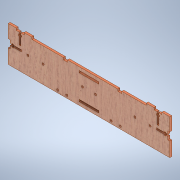
# Autodesk Inventor part: зад
Saved by Autodesk Inventor 2020 (Build 240168000, 168)
## iProperties
Created: 2025-01-17
Part Number: зад
Material: Дерево (орех)
Document SubType Name: ЛистМат
Designer: frozj
Density: 0.55 g/cm^3
Sheet Metal Rule: По умолчанию_мм
Appearance: Орех — натуральный — полированный
Author: frozj
Autodesk Inventor part; units mm, degrees
ref_plane "YZ Plane" through (0, 0, 0) normal (1, 0, 0) x (0, 1, 0)
ref_plane "XZ Plane" through (0, 0, 0) normal (0, 1, 0) x (-1, 0, 0)
ref_plane "XY Plane" through (0, 0, 0) normal (0, 0, 1) x (1, 0, 0)
sketch "Эскиз1" plane through (0, 0, 0) normal (0, 0, 1) x (1, 0, 0)
  line L0 (125, -28.5) -> (-125, -28.5)
  line L1 (-125, -28.5) -> (-125, 28.5)
  line L2 (-125, 28.5) -> (125, 28.5)
  line L3 (125, 28.5) -> (125, -28.5)
  line L4 (125, -28.5) -> (-125, 28.5) construction
  line L5 (-125, -28.5) -> (125, 28.5) construction
  line L6 (-125, 28.5) -> (125, 28.5)
  line L7 (125, 11.5) -> (-125, 11.5)
  line L8 (-125, 11.5) -> (-125, 28.5)
  line L9 (-125, 11.5) -> (125, 11.5)
  line L10 (125, 11.5) -> (125, -8.5)
  line L11 (125, -8.5) -> (-125, -8.5)
  line L12 (-125, -8.5) -> (-125, 11.5)
  line L13 (-125, -8.5) -> (125, -8.5)
  line L14 (125, -8.5) -> (125, -25.5)
  line L15 (125, -25.5) -> (-125, -25.5)
  line L16 (-125, -25.5) -> (-125, -8.5)
  line L17 (-125, 28.5) -> (125, 28.5)
  line L18 (125, 25.5) -> (-125, 25.5)
  line L19 (-125, 25.5) -> (-125, 28.5)
  line L20 (-125, 28.5) -> (-111, 28.5)
  line L21 (-111, 28.5) -> (-111, 25.5)
  line L22 (-111, 25.5) -> (-125, 25.5)
  line L23 (-125, 25.5) -> (-125, 28.5)
  line L24 (-111, 25.5) -> (-99, 25.5)
  line L25 (-99, 25.5) -> (-99, 28.5)
  line L26 (-99, 28.5) -> (-111, 28.5)
  line L27 (-111, 28.5) -> (-111, 25.5)
  line L28 (-99, 28.5) -> (-87, 28.5)
  line L29 (-87, 28.5) -> (-87, 25.5)
  line L30 (-87, 25.5) -> (-99, 25.5)
  line L31 (-99, 25.5) -> (-99, 28.5)
  line L32 (-111, 28.5) -> (-106.35, 28.5)
  line L33 (-106.35, 28.5) -> (-103.65, 28.5)
  line L34 (-103.65, 28.5) -> (-103.65, 8.5)
  line L35 (-103.65, 8.5) -> (-106.35, 8.5)
  line L36 (-106.35, 8.5) -> (-106.35, 28.5)
  line L37 (-106.35, 25.5) -> (-107.45, 25.5)
  line L38 (-107.45, 22.5) -> (-106.35, 22.5)
  line L39 (-106.35, 22.5) -> (-106.35, 25.5)
  line L40 (-107.45, 22.5) -> (-102.55, 22.5)
  line L41 (-102.55, 22.5) -> (-102.55, 20.6)
  line L42 (-102.55, 20.6) -> (-107.45, 20.6)
  line L43 (-107.45, 20.6) -> (-107.45, 22.5)
  line L44 (125, -28.5) -> (125, 28.5)
  line L45 (111, 28.5) -> (111, 25.5)
  line L46 (99, 25.5) -> (99, 28.5)
  line L47 (87, 28.5) -> (87, 25.5)
  line L48 (103.65, 28.5) -> (103.65, 8.5)
  line L49 (103.65, 8.5) -> (106.35, 8.5)
  line L50 (106.35, 8.5) -> (106.35, 28.5)
  line L51 (106.35, 22.5) -> (106.35, 25.5)
  line L52 (107.45, 22.5) -> (102.55, 22.5)
  line L53 (102.55, 22.5) -> (102.55, 20.6)
  line L54 (102.55, 20.6) -> (107.45, 20.6)
  line L55 (107.45, 20.6) -> (107.45, 22.5)
  line L56 (-125, 11.5) -> (-96, 11.5)
  line L57 (-96, 11.5) -> (-96, -8.5)
  line L58 (-96, -8.5) -> (-125, -8.5)
  line L59 (-125, -8.5) -> (-125, 11.5)
  line L60 (-96, -8.5) -> (-67, -8.5)
  line L61 (-67, -8.5) -> (-67, 11.5)
  line L62 (-67, 11.5) -> (-96, 11.5)
  line L63 (-96, 11.5) -> (-96, -8.5)
  line L64 (-96, 1.5) -> (-93, 1.5)
  line L65 (-67, 1.5) -> (-70, 1.5)
  circle A0 centre (-70, 1.5) radius 1.5
  circle A1 centre (-93, 1.5) radius 1.5
  circle A2 centre (70, 1.5) radius 1.5
  circle A3 centre (93, 1.5) radius 1.5
  line L66 (-125, 28.5) -> (-122, 28.5)
  line L67 (-126, 8.5) -> (-125, 28.5)
  line L68 (-126, -3.5) -> (-126, 8.5)
  line L69 (-126, 1.15) -> (-126, 3.85)
  line L70 (-125, 28.5) -> (-123, 28.5)
  line L71 (-123, 28.5) -> (-123, 8.5)
  line L72 (-123, 8.5) -> (-125, 8.5)
  line L73 (-125, 8.5) -> (-125, 28.5)
  line L74 (-123, 8.5) -> (-126, 8.5)
  line L75 (-126, 8.5) -> (-126, -3.5)
  line L76 (-126, -3.5) -> (-123, -3.5)
  line L77 (-123, -3.5) -> (-123, 8.5)
  line L78 (-123, 28.5) -> (-120, 28.5)
  line L79 (-120, 28.5) -> (-120, -3.5)
  line L80 (-120, -3.5) -> (-123, -3.5)
  line L81 (-123, -3.5) -> (-123, 28.5)
  line L82 (-123, 8.5) -> (-120, 8.5)
  line L83 (-120, 8.5) -> (-120, -3.5)
  line L84 (-120, -3.5) -> (-123, -3.5)
  line L85 (-123, -3.5) -> (-123, 8.5)
  line L86 (-123, 8.5) -> (-123, 3.85)
  line L87 (-123, 3.85) -> (-103, 3.85)
  line L88 (-103, 3.85) -> (-103, 1.15)
  line L89 (-103, 1.15) -> (-123, 1.15)
  line L90 (-123, 1.15) -> (-123, 3.85)
  line L91 (-120, 1.15) -> (-117, 1.15)
  line L92 (-117, 1.15) -> (-117, 0.05)
  line L93 (-117, 0.05) -> (-120, 0.05)
  line L94 (-120, 0.05) -> (-120, 1.15)
  line L95 (-117, 0.05) -> (-115.1, 0.05)
  line L96 (-115.1, 0.05) -> (-115.1, 4.95)
  line L97 (-115.1, 4.95) -> (-117, 4.95)
  line L98 (-117, 4.95) -> (-117, 0.05)
  line L99 (123, 3.85) -> (103, 3.85)
  line L100 (103, 3.85) -> (103, 1.15)
  line L101 (103, 1.15) -> (123, 1.15)
  line L102 (120, 1.15) -> (117, 1.15)
  line L103 (117, 0.05) -> (115.1, 0.05)
  line L104 (115.1, 0.05) -> (115.1, 4.95)
  line L105 (115.1, 4.95) -> (117, 4.95)
  line L106 (117, 4.95) -> (117, 0.05)
  line L107 (126, -3.5) -> (123, -3.5)
  line L108 (120, 28.5) -> (120, -3.5)
  line L109 (120, -3.5) -> (123, -3.5)
  line L110 (123, -3.5) -> (123, 28.5)
  line L111 (123, 8.5) -> (125, 8.5)
  line L112 (123, 8.5) -> (120, 8.5)
  line L113 (-123, -3.5) -> (-125, -3.5)
  line L114 (-125, -3.5) -> (-125, -28.5)
  line L115 (-125, -28.5) -> (-123, -28.5)
  line L116 (-123, -28.5) -> (-123, -3.5)
  line L117 (123, -3.5) -> (125, -3.5)
  line L118 (125, -3.5) -> (125, -28.5)
  line L119 (125, -28.5) -> (123, -28.5)
  line L120 (123, -28.5) -> (123, -3.5)
  line L121 (-67, -8.5) -> (-14.5, -8.5)
  line L122 (-14.5, -28.5) -> (-67, -28.5)
  line L123 (-40.75, -28.5) -> (-33.75, -28.5)
  circle A4 centre (-33.75, -21.5) radius 1.5
  circle A5 centre (-47.75, -21.5) radius 1.5
  circle A6 centre (33.75, -21.5) radius 1.5
  circle A7 centre (47.75, -21.5) radius 1.5
  line L124 (-33.75, -25.5) -> (-47.75, -25.5)
  line L125 (-47.75, -28.5) -> (-33.75, -28.5)
  line L126 (-40.75, -28.5) -> (-28.75, -28.5)
  line L127 (-28.75, -28.5) -> (-28.75, -25.5)
  line L128 (-28.75, -25.5) -> (-40.75, -25.5)
  line L129 (-40.75, -28.5) -> (-52.75, -28.5)
  line L130 (-52.75, -28.5) -> (-52.75, -25.5)
  line L131 (-52.75, -25.5) -> (-40.75, -25.5)
  line L132 (-40.75, -25.5) -> (-40.75, -28.5)
  line L133 (28.75, -28.5) -> (28.75, -25.5)
  line L134 (52.75, -28.5) -> (52.75, -25.5)
  line L135 (52.5, -17.5) -> (-52.5, -17.5)
  line L136 (-52.5, -17.5) -> (-52.5, 17.5)
  line L137 (-52.5, 17.5) -> (52.5, 17.5)
  line L138 (52.5, 17.5) -> (52.5, -17.5)
  line L139 (52.5, -17.5) -> (-52.5, 17.5) construction
  line L140 (-52.5, -17.5) -> (52.5, 17.5) construction
  line L141 (15, 14.5) -> (-15, 14.5)
  line L142 (-15, 14.5) -> (-15, 20.5)
  line L143 (-15, 20.5) -> (15, 20.5)
  line L144 (15, 20.5) -> (15, 14.5)
  line L145 (15, 14.5) -> (-15, 20.5) construction
  line L146 (-15, 14.5) -> (15, 20.5) construction
  line L147 (15, -20.5) -> (-15, -20.5)
  line L148 (-15, -20.5) -> (-15, -14.5)
  line L149 (-15, -14.5) -> (15, -14.5)
  line L150 (15, -14.5) -> (15, -20.5)
  line L151 (15, -20.5) -> (-15, -14.5) construction
  line L152 (-15, -20.5) -> (15, -14.5) construction
  line L153 (0, 0) -> (-36, 0)
  line L154 (-36, 0) -> (-36, 28.5)
  line L155 (-36, 28.5) -> (0, 28.5)
  line L156 (0, 28.5) -> (0, 0)
  line L157 (0, 0) -> (47, 0)
  line L158 (47, 0) -> (47, 28.5)
  line L159 (47, 28.5) -> (0, 28.5)
  line L160 (0, 28.5) -> (0, 0)
  line L161 (-36, 28.5) -> (-33, 28.5)
  line L162 (-33, 28.5) -> (-33, 25.5)
  line L163 (-33, 25.5) -> (-36, 25.5)
  line L164 (-36, 25.5) -> (-36, 28.5)
  line L165 (-36, 28.5) -> (-39, 28.5)
  line L166 (-39, 28.5) -> (-39, 25.5)
  line L167 (-39, 25.5) -> (-36, 25.5)
  line L168 (-36, 25.5) -> (-36, 28.5)
  line L169 (47, 28.5) -> (44, 28.5)
  line L170 (44, 28.5) -> (44, 25.5)
  line L171 (44, 25.5) -> (47, 25.5)
  line L172 (47, 25.5) -> (47, 28.5)
  line L173 (47, 28.5) -> (50, 28.5)
  line L174 (50, 28.5) -> (50, 25.5)
  line L175 (50, 25.5) -> (47, 25.5)
  line L176 (47, 25.5) -> (47, 28.5)
  line L177 (-39, 25.5) -> (-33, 25.5)
  line L178 (-33, 25.5) -> (-33, 22.5)
  line L179 (-33, 22.5) -> (-39, 22.5)
  line L180 (-39, 22.5) -> (-39, 25.5)
  line L181 (50, 25.5) -> (44, 25.5)
  line L182 (44, 25.5) -> (44, 22.5)
  line L183 (44, 22.5) -> (50, 22.5)
  line L184 (50, 22.5) -> (50, 25.5)
  line L185 (-70, 1.5) -> (70, 1.5)
  line L186 (0, 1.5) -> (10, 1.5)
  line L187 (10, 1.5) -> (-10, 1.5)
  circle A8 centre (-10, 1.5) radius 1.5
  circle A9 centre (10, 1.5) radius 1.5
  point P0 (106.35, 20.6)
  point P1 (103.65, 20.6)
  point P2 (103.65, 22.5)
  point P3 (103.65, 25.5)
  point P4 (-103.65, 25.5)
  point P5 (-103.65, 22.5)
  point P6 (-103.65, 20.6)
  point P7 (-106.35, 20.6)
  point P8 (106.35, 11.5)
  point P9 (103.65, 11.5)
  point P10 (-103.65, 11.5)
  point P11 (-106.35, 11.5)
  point P12 (-120, 3.85)
  point P13 (-117, 3.85)
  point P14 (-115.1, 3.85)
  point P15 (-115.1, 1.15)
  point P16 (-117, 1.15)
  point P17 (-120, 1.15)
  point P18 (115.1, 1.15)
  point P19 (115.1, 3.85)
  point P20 (117, 3.85)
  point P21 (120, 3.85)
  point P22 (120, 11.5)
  point P23 (-123, -28.5)
  point P24 (123, 28.5)
  point P25 (0, 17.5)
  point P26 (0, -17.5)
  point P27 (-15, 17.5)
  point P28 (15, 17.5)
  point P29 (-15, -17.5)
  point P30 (15, -17.5)
  point P31 (-123, -25.5)
  point P32 (123, -25.5)
  dimension "d0" = 250
  dimension "d1" = 57
  dimension "d2" = 17
  dimension "d3" = 20
  dimension "d4" = 17
  dimension "d8" = 3
  dimension "d9" = 14
  dimension "d10" = 12
  dimension "d11" = 12
  dimension "d12" = 4.65
  dimension "d14" = 20
  dimension "d15" = 1.1
  dimension "d16" = 3
  dimension "d17" = 4.9
  dimension "d18" = 1.9
  dimension "d23" = 29
  dimension "d24" = 29
  dimension "d25" = 3
  dimension "d26" = 3
  dimension "d27" = 3
  dimension "d31" = 4.65
  dimension "d37" = 2
  dimension "d38" = 20
  dimension "d39" = 12
  dimension "d40" = 3
  dimension "d41" = 20
  dimension "d42" = 2.7
  dimension "d43" = 3
  dimension "d44" = 1.1
  dimension "d45" = 1.9
  dimension "d46" = 4.9
  dimension "d49" = 3
  dimension "d50" = 12
  dimension "d51" = 12
  dimension "d52" = 105
  dimension "d53" = 35
  dimension "d54" = 30
  dimension "d55" = 6
  dimension "d56" = 30
  dimension "d57" = 6
  dimension "d58" = 33.75
  dimension "d59" = 36
  dimension "d60" = 47
  dimension "d61" = 3
  dimension "d62" = 3
  dimension "d63" = 3
  dimension "d64" = 3
  dimension "d65" = 96
  dimension "d66" = 10
  dimension "d67" = 20
  dimension "d68" = 3
  dimension "d69" = 3
  constraints: 376 end point, 68 parallel, 40 horizontal, 33 point on line, 32 perpendicular, 13 midpoint, 10 centre point, 4 coincident
  measures "d0" distance of L1.end L2.end
  measures "d1" distance of L0.end L1.end
  measures "d2" distance of L6.end L7.start
  measures "d3" distance of L9.end L10.end
  measures "d4" distance of L13.end L14.end
  measures "d8" distance of L17.end L18.start
  measures "d9" distance of L21.end L22.end
  measures "d10" distance of L26.end L25.end
  measures "d11" distance of L29.end L30.end
  measures "d12" distance of L26.end L32.end
  measures "d14" distance of L33.end L34.end
  measures "d15" distance of L38.end L38.start
  measures "d16" distance of L38.start L37.end
  measures "d17" distance of L41.end L42.end
  measures "d18" distance of L40.end L41.end
  measures "d23" distance of L57.end L58.end
  measures "d24" distance of L62.end L61.end
  measures "d25" distance of L65.start L65.end
  measures "d26" diameter of A0
  measures "d27" diameter of A1
  measures "d31" distance of L67.start L69.end
  measures "d37" distance of L71.end L72.end
  measures "d38" distance of L70.end L71.end
  measures "d39" distance of L68.start L74.end
  measures "d40" distance of L79.end L80.end
  measures "d41" distance of L88.end L89.end
  measures "d42" distance of L87.end L88.end
  measures "d43" distance of L92.end L93.end
  measures "d44" distance of L91.end L92.end
  measures "d45" distance of L97.end L96.end
  measures "d46" distance of L96.end L95.end
  measures "d49" diameter of A4
  measures "d50" distance of L128.end L127.end
  measures "d51" distance of L130.end L131.end
  measures "d52" distance of L136.end L137.end
  measures "d53" distance of L135.end L136.end
  measures "d54" distance of L142.end L143.end
  measures "d55" distance of L141.end L142.end
  measures "d56" distance of L148.end L149.end
  measures "d57" distance of L147.end L148.end
  measures "d58" horizontal distance of A4.centre L153.start
  measures "d59" distance of L154.end L155.end
  measures "d60" distance of L159.end L158.end
  measures "d61" distance of L162.end L163.end
  measures "d62" distance of L167.end L166.end
  measures "d63" distance of L171.end L170.end
  measures "d64" distance of L174.end L175.end
  measures "d65" distance from line of L153.start L57
  measures "d66" distance of L186.start L186.end
  measures "d67" distance of L186.end L187.end
  measures "d68" diameter of A8
  measures "d69" diameter of A9
extrude "Выдавливание1" add sketch "Эскиз1" along normal blind 3 contours L15 L116 L11 L136 L135 L148 L147 L150 L138 L120 | L11 L138 L7 L48 L49 L50 L108 L99 L106 L105 L104 L100 L101 L103 L109 L120 | L138 L135 L150 L149 L148 L136 L11 | L11 L136 L185 L154 L153 L157 L158 L138 | L185 L158 L7 L138 | L112 L108 L7 L110 | L11 L61 L185 L136 | L138 L137 L158 L183 L184 L18 L48 L52 L53 L54 L7 | L7 L158 L137 L138 | L185 A9 L156 L7 L158 | L158 L157 A9 L185 | L135 L148 L149 L150 | L7 L108 L18 L110 | L11 L57 L7 L61 | L185 L61 L7 L136 | L136 L7 L154 L185 | L7 L156 L141 L144 L137 L158 | L18 L108 L2 L110 | L7 L50 L54 L55 L52 L18 L108 | L11 L116 L80 L79 L93 L95 L96 L89 L88 L87 L97 L98 L7 L36 L35 L34 L57 | L136 L137 L154 L7 | L7 L34 L42 L41 L40 L18 L180 L179 L154 L137 L136 | L185 A8 L153 L154 | L154 L7 L156 L185 A8 | L7 L154 L137 L142 L141 L156 | L137 L144 L143 L156 L18 L182 L183 L158 | L157 L156 L185 A9 | L18 L45 L2 L108 | L156 L137 L144 L141 | L141 L142 L137 L156 | L156 L153 A8 L185 | L154 L179 L178 L18 L156 L143 L142 L137 | L18 L47 L2 L46 | L89 L92 L93 L79 | L7 L79 L18 L36 L38 L43 L42 | L71 L7 L79 L82 | L7 L71 L18 L79 | L79 L2 L21 L18 | L18 L71 L2 L79 | L18 L25 L2 L29
equation "\"Радиус_гибки\" = Толщина"
equation "\"Ширина_просечки\" = Толщина"
equation "\"Глубина_просечки\" = 0.5 * Толщина"
equation "\"Размер_просечки\" = 4 * Толщина"
equation "\"Мин_остаток\" = 2 * Толщина"
equation "\"Радиус_перехода\" = Радиус_гибки"
equation "\"Радиус_Якоби\" = Радиус_гибки"
equation "\"Размер_зазора\" = Толщина"
equation "\"Толщина\" = 0.5"
